Autodesk Inventor part; units mm, degrees
(part 5 of 7)
  arc A234 (19.9489, -1.9822) -> (19.5895, -1.8197) centre (17.1307, -7.7369) ccw projected
  arc A235 (20.3804, -2.2111) -> (19.9489, -1.9822) centre (16.6119, -8.7963) ccw projected
  arc A236 (20.3335, -2.6078) -> (20.3804, -2.2111) centre (0, 0) ccw projected
  arc A237 (19.8604, -2.7295) -> (20.3335, -2.6078) centre (18.2064, 4.6753) ccw projected
  arc A238 (19.473, -2.8036) -> (19.8604, -2.7295) centre (18.4635, 3.5241) ccw projected
  arc A239 (19.1652, -2.8435) -> (19.473, -2.8036) centre (18.6425, 2.4025) ccw projected
  arc A240 (19.1059, -3.2181) -> (19.1652, -2.8435) centre (0, 0) ccw projected
  arc A241 (19.3863, -3.3511) -> (19.1059, -3.2181) centre (16.9876, -8.0457) ccw projected
  arc A242 (19.7318, -3.5413) -> (19.3863, -3.3511) centre (16.4708, -9.0571) ccw projected
  arc A243 (20.1441, -3.8033) -> (19.7318, -3.5413) centre (15.8705, -10.0726) ccw projected
  arc A244 (20.0662, -4.1951) -> (20.1441, -3.8033) centre (0, 0) ccw projected
  arc A245 (19.585, -4.2793) -> (20.0662, -4.1951) centre (18.517, 3.2324) ccw projected
  arc A246 (19.193, -4.3228) -> (19.585, -4.2793) centre (18.6831, 2.0646) ccw projected
  arc A247 (18.883, -4.3384) -> (19.193, -4.3228) centre (18.7735, 0.9324) ccw projected
  arc A248 (18.7945, -4.7072) -> (18.883, -4.3384) centre (0, 0) ccw projected
  arc A249 (19.0636, -4.8618) -> (18.7945, -4.7072) centre (16.304, -9.3537) ccw projected
  arc A250 (19.3932, -5.0785) -> (19.0636, -4.8618) centre (15.7095, -10.3215) ccw projected
  arc A251 (19.7836, -5.372) -> (19.3932, -5.0785) centre (15.0313, -11.2867) ccw projected
  arc A252 (19.6752, -5.7565) -> (19.7836, -5.372) centre (0, 0) ccw projected
  arc A253 (19.1889, -5.8028) -> (19.6752, -5.7565) centre (18.7136, 1.7696) ccw projected
  arc A254 (18.7947, -5.8154) -> (19.1889, -5.8028) centre (18.7875, 0.5924) ccw projected
  arc A255 (18.4844, -5.8066) -> (18.7947, -5.8154) centre (18.7888, -0.5434) ccw projected
  arc A256 (18.3672, -6.1673) -> (18.4844, -5.8066) centre (0, 0) ccw projected
  arc A257 (18.6234, -6.3425) -> (18.3672, -6.1673) centre (15.5199, -10.6041) ccw projected
  arc A258 (18.9349, -6.5844) -> (18.6234, -6.3425) centre (14.8512, -11.5222) ccw projected
  arc A259 (19.3011, -6.9077) -> (18.9349, -6.5844) centre (14.0994, -12.4312) ccw projected
  arc A260 (19.1629, -7.2825) -> (19.3011, -6.9077) centre (0, 0) ccw projected
  arc A261 (18.6745, -7.2904) -> (19.1629, -7.2825) centre (18.7947, 0.2959) ccw projected
  arc A262 (18.2805, -7.272) -> (18.6745, -7.2904) centre (18.776, -0.8835) ccw projected
  arc A263 (17.9719, -7.2389) -> (18.2805, -7.272) centre (18.6882, -2.0159) ccw projected
  arc A264 (17.8267, -7.5893) -> (17.9719, -7.2389) centre (0, 0) ccw projected
  arc A265 (18.0684, -7.7842) -> (17.8267, -7.5893) centre (14.64, -11.7891) ccw projected
  arc A266 (18.36, -8.0497) -> (18.0684, -7.7842) centre (13.9014, -12.6519) ccw projected
  arc A267 (18.6997, -8.4007) -> (18.36, -8.0497) centre (13.0806, -13.4991) ccw projected
  arc A268 (18.5324, -8.7635) -> (18.6997, -8.4007) centre (0, 0) ccw projected
  arc A269 (18.0449, -8.7331) -> (18.5324, -8.7635) centre (18.76, -1.1796) ccw projected
  arc A270 (17.6536, -8.6839) -> (18.0449, -8.7331) centre (18.6488, -2.3539) ccw projected
  arc A271 (17.3485, -8.6267) -> (17.6536, -8.6839) centre (18.4724, -3.476) ccw projected
  arc A272 (17.1763, -8.9646) -> (17.3485, -8.6267) centre (0, 0) ccw projected
  arc A273 (17.4019, -9.1778) -> (17.1763, -8.9646) centre (13.6699, -12.9014) ccw projected
  arc A274 (17.6718, -9.4654) -> (17.4019, -9.1778) centre (12.8659, -13.7036) ccw projected
  arc A275 (17.9829, -9.842) -> (17.6718, -9.4654) centre (11.9812, -14.4838) ccw projected
  arc A276 (17.7877, -10.1905) -> (17.9829, -9.842) centre (0, 0) ccw projected
  arc A277 (17.3041, -10.122) -> (17.7877, -10.1905) centre (18.6096, -2.6478) ccw projected
  arc A278 (16.9178, -10.0422) -> (17.3041, -10.122) centre (18.4067, -3.8099) ccw projected
  arc A279 (16.6182, -9.9612) -> (16.9178, -10.0422) centre (18.1428, -4.9146) ccw projected
  arc A280 (16.42, -10.2846) -> (16.6182, -9.9612) centre (0, 0) ccw projected
  arc A281 (16.6282, -10.5148) -> (16.42, -10.2846) centre (12.6156, -13.9341) ccw projected
  arc A282 (16.8747, -10.8227) -> (16.6282, -10.5148) centre (11.7511, -14.6708) ccw projected
  arc A283 (17.1553, -11.2226) -> (16.8747, -10.8227) centre (10.8078, -15.3792) ccw projected
  arc A284 (16.9334, -11.5547) -> (17.1553, -11.2226) centre (0, 0) ccw projected
  arc A285 (16.4566, -11.4485) -> (16.9334, -11.5547) centre (18.3445, -4.0998) ccw projected
  arc A286 (16.0778, -11.3386) -> (16.4566, -11.4485) centre (18.051, -5.2423) ccw projected
  arc A287 (15.7854, -11.2344) -> (16.0778, -11.3386) centre (17.7012, -6.3229) ccw projected
  arc A288 (15.5625, -11.5412) -> (15.7854, -11.2344) centre (0, 0) ccw projected
  arc A289 (15.752, -11.7871) -> (15.5625, -11.5412) centre (11.4834, -14.881) ccw projected
  arc A290 (15.9735, -12.1134) -> (15.752, -11.7871) centre (10.5638, -15.5476) ccw projected
  arc A291 (16.2219, -12.534) -> (15.9735, -12.1134) centre (9.5679, -16.1798) ccw projected
  arc A292 (15.9746, -12.8477) -> (16.2219, -12.534) centre (0, 0) ccw projected
  arc A293 (15.5076, -12.7043) -> (15.9746, -12.8477) centre (17.9663, -5.5264) ccw projected
  arc A294 (15.1386, -12.5651) -> (15.5076, -12.7043) centre (17.5841, -6.6424) ccw projected
  arc A295 (14.8553, -12.4383) -> (15.1386, -12.5651) centre (17.1506, -7.6922) ccw projected
  arc A296 (14.609, -12.7266) -> (14.8553, -12.4383) centre (0, 0) ccw projected
  arc A297 (14.7786, -12.9866) -> (14.609, -12.7266) centre (10.2805, -15.7361) ccw projected
  arc A298 (14.9739, -13.3293) -> (14.7786, -12.9866) centre (9.3114, -16.3285) ccw projected
  arc A299 (15.1885, -13.7681) -> (14.9739, -13.3293) centre (8.2689, -16.8806) ccw projected
  arc A300 (14.9173, -14.0614) -> (15.1885, -13.7681) centre (0, 0) ccw projected
  arc A301 (14.463, -13.8819) -> (14.9173, -14.0614) centre (17.4773, -6.919) ccw projected
  arc A302 (14.1061, -13.7141) -> (14.463, -13.8819) centre (17.0087, -8.0015) ccw projected
  arc A303 (13.8336, -13.5655) -> (14.1061, -13.7141) centre (16.4942, -9.0141) ccw projected
  arc A304 (13.5655, -13.8336) -> (13.8336, -13.5655) centre (0, 0) ccw projected
  arc A305 (13.7141, -14.1061) -> (13.5655, -13.8336) centre (9.0141, -16.4942) ccw projected
  arc A306 (13.8819, -14.463) -> (13.7141, -14.1061) centre (8.0015, -17.0087) ccw projected
  arc A307 (14.0614, -14.9173) -> (13.8819, -14.463) centre (6.919, -17.4773) ccw projected
  arc A308 (13.7681, -15.1885) -> (14.0614, -14.9173) centre (0, 0) ccw projected
  arc A309 (13.3293, -14.9739) -> (13.7681, -15.1885) centre (16.8806, -8.2689) ccw projected
  arc A310 (12.9866, -14.7786) -> (13.3293, -14.9739) centre (16.3285, -9.3114) ccw projected
  arc A311 (12.7266, -14.609) -> (12.9866, -14.7786) centre (15.7361, -10.2805) ccw projected
  arc A312 (12.4383, -14.8553) -> (12.7266, -14.609) centre (0, 0) ccw projected
  arc A313 (12.5651, -15.1386) -> (12.4383, -14.8553) centre (7.6922, -17.1506) ccw projected
  arc A314 (12.7043, -15.5076) -> (12.5651, -15.1386) centre (6.6424, -17.5841) ccw projected
  arc A315 (12.8477, -15.9746) -> (12.7043, -15.5076) centre (5.5264, -17.9663) ccw projected
  arc A316 (12.534, -16.2219) -> (12.8477, -15.9746) centre (0, 0) ccw projected
  arc A317 (12.1134, -15.9735) -> (12.534, -16.2219) centre (16.1798, -9.5679) ccw projected
  arc A318 (11.7871, -15.752) -> (12.1134, -15.9735) centre (15.5476, -10.5638) ccw projected
  arc A319 (11.5412, -15.5625) -> (11.7871, -15.752) centre (14.881, -11.4834) ccw projected
  arc A320 (11.2344, -15.7854) -> (11.5412, -15.5625) centre (0, 0) ccw projected
  arc A321 (11.3386, -16.0778) -> (11.2344, -15.7854) centre (6.3229, -17.7012) ccw projected
  arc A322 (11.4485, -16.4566) -> (11.3386, -16.0778) centre (5.2423, -18.051) ccw projected
  arc A323 (11.5547, -16.9334) -> (11.4485, -16.4566) centre (4.0998, -18.3445) ccw projected
  arc A324 (11.2226, -17.1553) -> (11.5547, -16.9334) centre (0, 0) ccw projected
  arc A325 (10.8227, -16.8747) -> (11.2226, -17.1553) centre (15.3792, -10.8078) ccw projected
  arc A326 (10.5148, -16.6282) -> (10.8227, -16.8747) centre (14.6708, -11.7511) ccw projected
  arc A327 (10.2846, -16.42) -> (10.5148, -16.6282) centre (13.9341, -12.6156) ccw projected
  arc A328 (9.9612, -16.6182) -> (10.2846, -16.42) centre (0, 0) ccw projected
  arc A329 (10.0422, -16.9178) -> (9.9612, -16.6182) centre (4.9146, -18.1428) ccw projected
  arc A330 (10.122, -17.3041) -> (10.0422, -16.9178) centre (3.8099, -18.4067) ccw projected
  arc A331 (10.1905, -17.7877) -> (10.122, -17.3041) centre (2.6478, -18.6096) ccw projected
  arc A332 (9.842, -17.9829) -> (10.1905, -17.7877) centre (0, 0) ccw projected
  arc A333 (9.4654, -17.6718) -> (9.842, -17.9829) centre (14.4838, -11.9812) ccw projected
  arc A334 (9.1778, -17.4019) -> (9.4654, -17.6718) centre (13.7036, -12.8659) ccw projected
  arc A335 (8.9646, -17.1763) -> (9.1778, -17.4019) centre (12.9014, -13.6699) ccw projected
  arc A336 (8.6267, -17.3485) -> (8.9646, -17.1763) centre (0, 0) ccw projected
  arc A337 (8.6839, -17.6536) -> (8.6267, -17.3485) centre (3.476, -18.4724) ccw projected
  arc A338 (8.7331, -18.0449) -> (8.6839, -17.6536) centre (2.3539, -18.6488) ccw projected
  arc A339 (8.7635, -18.5324) -> (8.7331, -18.0449) centre (1.1796, -18.76) ccw projected
  arc A340 (8.4007, -18.6997) -> (8.7635, -18.5324) centre (0, 0) ccw projected
  arc A341 (8.0497, -18.36) -> (8.4007, -18.6997) centre (13.4991, -13.0806) ccw projected
  arc A342 (7.7842, -18.0684) -> (8.0497, -18.36) centre (12.6519, -13.9014) ccw projected
  arc A343 (7.5893, -17.8267) -> (7.7842, -18.0684) centre (11.7891, -14.64) ccw projected
  arc A344 (7.2389, -17.9719) -> (7.5893, -17.8267) centre (0, 0) ccw projected
  arc A345 (7.272, -18.2805) -> (7.2389, -17.9719) centre (2.0159, -18.6882) ccw projected
  arc A346 (7.2904, -18.6745) -> (7.272, -18.2805) centre (0.8835, -18.776) ccw projected
  arc A347 (7.2825, -19.1629) -> (7.2904, -18.6745) centre (-0.2959, -18.7947) ccw projected
  arc A348 (6.9077, -19.3011) -> (7.2825, -19.1629) centre (0, 0) ccw projected
  arc A349 (6.5844, -18.9349) -> (6.9077, -19.3011) centre (12.4312, -14.0994) ccw projected
  arc A350 (6.3425, -18.6234) -> (6.5844, -18.9349) centre (11.5222, -14.8512) ccw projected
  arc A351 (6.1673, -18.3672) -> (6.3425, -18.6234) centre (10.6041, -15.5199) ccw projected
  arc A352 (5.8066, -18.4844) -> (6.1673, -18.3672) centre (0, 0) ccw projected
  arc A353 (5.8154, -18.7947) -> (5.8066, -18.4844) centre (0.5434, -18.7888) ccw projected
  arc A354 (5.8028, -19.1889) -> (5.8154, -18.7947) centre (-0.5924, -18.7875) ccw projected
  arc A355 (5.7565, -19.6752) -> (5.8028, -19.1889) centre (-1.7696, -18.7136) ccw projected
  arc A356 (5.372, -19.7836) -> (5.7565, -19.6752) centre (0, 0) ccw projected
  arc A357 (5.0785, -19.3932) -> (5.372, -19.7836) centre (11.2867, -15.0313) ccw projected
  arc A358 (4.8618, -19.0636) -> (5.0785, -19.3932) centre (10.3215, -15.7095) ccw projected
  arc A359 (4.7072, -18.7945) -> (4.8618, -19.0636) centre (9.3537, -16.304) ccw projected
  arc A360 (4.3384, -18.883) -> (4.7072, -18.7945) centre (0, 0) ccw projected
  arc A361 (4.3228, -19.193) -> (4.3384, -18.883) centre (-0.9324, -18.7735) ccw projected
  arc A362 (4.2793, -19.585) -> (4.3228, -19.193) centre (-2.0646, -18.6831) ccw projected
  arc A363 (4.1951, -20.0662) -> (4.2793, -19.585) centre (-3.2324, -18.517) ccw projected
  arc A364 (3.8033, -20.1441) -> (4.1951, -20.0662) centre (0, 0) ccw projected
  arc A365 (3.5413, -19.7318) -> (3.8033, -20.1441) centre (10.0726, -15.8705) ccw projected
  arc A366 (3.3511, -19.3863) -> (3.5413, -19.7318) centre (9.0571, -16.4708) ccw projected
  arc A367 (3.2181, -19.1059) -> (3.3511, -19.3863) centre (8.0457, -16.9876) ccw projected
  arc A368 (2.8435, -19.1652) -> (3.2181, -19.1059) centre (0, 0) ccw projected
  arc A369 (2.8036, -19.473) -> (2.8435, -19.1652) centre (-2.4025, -18.6425) ccw projected
  arc A370 (2.7295, -19.8604) -> (2.8036, -19.473) centre (-3.5241, -18.4635) ccw projected
  arc A371 (2.6078, -20.3335) -> (2.7295, -19.8604) centre (-4.6753, -18.2064) ccw projected
  arc A372 (2.2111, -20.3804) -> (2.6078, -20.3335) centre (0, 0) ccw projected
  arc A373 (1.9822, -19.9489) -> (2.2111, -20.3804) centre (8.7963, -16.6119) ccw projected
  arc A374 (1.8197, -19.5895) -> (1.9822, -19.9489) centre (7.7369, -17.1307) ccw projected
  arc A375 (1.7091, -19.2995) -> (1.8197, -19.5895) centre (6.6881, -17.5665) ccw projected
  arc A376 (1.331, -19.3292) -> (1.7091, -19.2995) centre (0, 0) ccw projected
  arc A377 (1.2671, -19.633) -> (1.331, -19.3292) centre (-3.8577, -18.3965) ccw projected
  arc A378 (1.1629, -20.0133) -> (1.2671, -19.633) centre (-4.9618, -18.1301) ccw projected
  arc A379 (1.0044, -20.4754) -> (1.1629, -20.0133) centre (-6.0894, -17.7834) ccw projected
  arc A380 (0.6052, -20.4911) -> (1.0044, -20.4754) centre (0, 0) ccw projected
  arc A381 (0.4109, -20.0429) -> (0.6052, -20.4911) centre (7.4658, -17.2508) ccw projected
  arc A382 (0.2771, -19.6719) -> (0.4109, -20.0429) centre (6.369, -17.6849) ccw projected
  arc A383 (0.1896, -19.3741) -> (0.2771, -19.6719) centre (5.2892, -18.0371) ccw projected
  arc A384 (-0.1896, -19.3741) -> (0.1896, -19.3741) centre (0, 0) ccw projected
  arc A385 (-0.2771, -19.6719) -> (-0.1896, -19.3741) centre (-5.2892, -18.0371) ccw projected
  arc A386 (-0.4109, -20.0429) -> (-0.2771, -19.6719) centre (-6.369, -17.6849) ccw projected
  arc A387 (-0.6052, -20.4911) -> (-0.4109, -20.0429) centre (-7.4658, -17.2508) ccw projected
  arc A388 (-1.0044, -20.4754) -> (-0.6052, -20.4911) centre (0, 0) ccw projected
  arc A389 (-1.1629, -20.0133) -> (-1.0044, -20.4754) centre (6.0894, -17.7834) ccw projected
  arc A390 (-1.2671, -19.633) -> (-1.1629, -20.0133) centre (4.9618, -18.1301) ccw projected
  arc A391 (-1.331, -19.3292) -> (-1.2671, -19.633) centre (3.8577, -18.3965) ccw projected
  arc A392 (-1.7091, -19.2995) -> (-1.331, -19.3292) centre (0, 0) ccw projected
  arc A393 (-1.8197, -19.5895) -> (-1.7091, -19.2995) centre (-6.6881, -17.5665) ccw projected
  arc A394 (-1.9822, -19.9489) -> (-1.8197, -19.5895) centre (-7.7369, -17.1307) ccw projected
  arc A395 (-2.2111, -20.3804) -> (-1.9822, -19.9489) centre (-8.7963, -16.6119) ccw projected
  arc A396 (-2.6078, -20.3335) -> (-2.2111, -20.3804) centre (0, 0) ccw projected
  arc A397 (-2.7295, -19.8604) -> (-2.6078, -20.3335) centre (4.6753, -18.2064) ccw projected
  arc A398 (-2.8036, -19.473) -> (-2.7295, -19.8604) centre (3.5241, -18.4635) ccw projected
  arc A399 (-2.8435, -19.1652) -> (-2.8036, -19.473) centre (2.4025, -18.6425) ccw projected
  arc A400 (-3.2181, -19.1059) -> (-2.8435, -19.1652) centre (0, 0) ccw projected
  arc A401 (-3.3511, -19.3863) -> (-3.2181, -19.1059) centre (-8.0457, -16.9876) ccw projected
  arc A402 (-3.5413, -19.7318) -> (-3.3511, -19.3863) centre (-9.0571, -16.4708) ccw projected
  arc A403 (-3.8033, -20.1441) -> (-3.5413, -19.7318) centre (-10.0726, -15.8705) ccw projected
  arc A404 (-4.1951, -20.0662) -> (-3.8033, -20.1441) centre (0, 0) ccw projected
  arc A405 (-4.2793, -19.585) -> (-4.1951, -20.0662) centre (3.2324, -18.517) ccw projected
  arc A406 (-4.3228, -19.193) -> (-4.2793, -19.585) centre (2.0646, -18.6831) ccw projected
  arc A407 (-4.3384, -18.883) -> (-4.3228, -19.193) centre (0.9324, -18.7735) ccw projected
  arc A408 (-4.7072, -18.7945) -> (-4.3384, -18.883) centre (0, 0) ccw projected
  arc A409 (-4.8618, -19.0636) -> (-4.7072, -18.7945) centre (-9.3537, -16.304) ccw projected
  arc A410 (-5.0785, -19.3932) -> (-4.8618, -19.0636) centre (-10.3215, -15.7095) ccw projected
  arc A411 (-5.372, -19.7836) -> (-5.0785, -19.3932) centre (-11.2867, -15.0313) ccw projected
  arc A412 (-5.7565, -19.6752) -> (-5.372, -19.7836) centre (0, 0) ccw projected
  arc A413 (-5.8028, -19.1889) -> (-5.7565, -19.6752) centre (1.7696, -18.7136) ccw projected
  arc A414 (-5.8154, -18.7947) -> (-5.8028, -19.1889) centre (0.5924, -18.7875) ccw projected
  arc A415 (-5.8066, -18.4844) -> (-5.8154, -18.7947) centre (-0.5434, -18.7888) ccw projected
  arc A416 (-6.1673, -18.3672) -> (-5.8066, -18.4844) centre (0, 0) ccw projected
  arc A417 (-6.3425, -18.6234) -> (-6.1673, -18.3672) centre (-10.6041, -15.5199) ccw projected
  arc A418 (-6.5844, -18.9349) -> (-6.3425, -18.6234) centre (-11.5222, -14.8512) ccw projected
  arc A419 (-6.9077, -19.3011) -> (-6.5844, -18.9349) centre (-12.4312, -14.0994) ccw projected
  arc A420 (-7.2825, -19.1629) -> (-6.9077, -19.3011) centre (0, 0) ccw projected
  arc A421 (-7.2904, -18.6745) -> (-7.2825, -19.1629) centre (0.2959, -18.7947) ccw projected
  arc A422 (-7.272, -18.2805) -> (-7.2904, -18.6745) centre (-0.8835, -18.776) ccw projected
  arc A423 (-7.2389, -17.9719) -> (-7.272, -18.2805) centre (-2.0159, -18.6882) ccw projected
  arc A424 (-7.5893, -17.8267) -> (-7.2389, -17.9719) centre (0, 0) ccw projected
  arc A425 (-7.7842, -18.0684) -> (-7.5893, -17.8267) centre (-11.7891, -14.64) ccw projected
  arc A426 (-8.0497, -18.36) -> (-7.7842, -18.0684) centre (-12.6519, -13.9014) ccw projected
  arc A427 (-8.4007, -18.6997) -> (-8.0497, -18.36) centre (-13.4991, -13.0806) ccw projected
  arc A428 (-8.7635, -18.5324) -> (-8.4007, -18.6997) centre (0, 0) ccw projected
  arc A429 (-8.7331, -18.0449) -> (-8.7635, -18.5324) centre (-1.1796, -18.76) ccw projected
  arc A430 (-8.6839, -17.6536) -> (-8.7331, -18.0449) centre (-2.3539, -18.6488) ccw projected
  arc A431 (-8.6267, -17.3485) -> (-8.6839, -17.6536) centre (-3.476, -18.4724) ccw projected
  arc A432 (-8.9646, -17.1763) -> (-8.6267, -17.3485) centre (0, 0) ccw projected
  arc A433 (-9.1778, -17.4019) -> (-8.9646, -17.1763) centre (-12.9014, -13.6699) ccw projected
  arc A434 (-9.4654, -17.6718) -> (-9.1778, -17.4019) centre (-13.7036, -12.8659) ccw projected
  arc A435 (-9.842, -17.9829) -> (-9.4654, -17.6718) centre (-14.4838, -11.9812) ccw projected
  arc A436 (-10.1905, -17.7877) -> (-9.842, -17.9829) centre (0, 0) ccw projected
  arc A437 (-10.122, -17.3041) -> (-10.1905, -17.7877) centre (-2.6478, -18.6096) ccw projected
  arc A438 (-10.0422, -16.9178) -> (-10.122, -17.3041) centre (-3.8099, -18.4067) ccw projected
  arc A439 (-9.9612, -16.6182) -> (-10.0422, -16.9178) centre (-4.9146, -18.1428) ccw projected
  arc A440 (-10.2846, -16.42) -> (-9.9612, -16.6182) centre (0, 0) ccw projected
  arc A441 (-10.5148, -16.6282) -> (-10.2846, -16.42) centre (-13.9341, -12.6156) ccw projected
  arc A442 (-10.8227, -16.8747) -> (-10.5148, -16.6282) centre (-14.6708, -11.7511) ccw projected
  arc A443 (-11.2226, -17.1553) -> (-10.8227, -16.8747) centre (-15.3792, -10.8078) ccw projected
  arc A444 (-11.5547, -16.9334) -> (-11.2226, -17.1553) centre (0, 0) ccw projected
  arc A445 (-11.4485, -16.4566) -> (-11.5547, -16.9334) centre (-4.0998, -18.3445) ccw projected
  arc A446 (-11.3386, -16.0778) -> (-11.4485, -16.4566) centre (-5.2423, -18.051) ccw projected
  arc A447 (-11.2344, -15.7854) -> (-11.3386, -16.0778) centre (-6.3229, -17.7012) ccw projected
  arc A448 (-11.5412, -15.5625) -> (-11.2344, -15.7854) centre (0, 0) ccw projected
  arc A449 (-11.7871, -15.752) -> (-11.5412, -15.5625) centre (-14.881, -11.4834) ccw projected
  arc A450 (-12.1134, -15.9735) -> (-11.7871, -15.752) centre (-15.5476, -10.5638) ccw projected
  arc A451 (-12.534, -16.2219) -> (-12.1134, -15.9735) centre (-16.1798, -9.5679) ccw projected
  arc A452 (-12.8477, -15.9746) -> (-12.534, -16.2219) centre (0, 0) ccw projected
  arc A453 (-12.7043, -15.5076) -> (-12.8477, -15.9746) centre (-5.5264, -17.9663) ccw projected
  arc A454 (-12.5651, -15.1386) -> (-12.7043, -15.5076) centre (-6.6424, -17.5841) ccw projected
  arc A455 (-12.4383, -14.8553) -> (-12.5651, -15.1386) centre (-7.6922, -17.1506) ccw projected
  arc A456 (-12.7266, -14.609) -> (-12.4383, -14.8553) centre (0, 0) ccw projected
  arc A457 (-12.9866, -14.7786) -> (-12.7266, -14.609) centre (-15.7361, -10.2805) ccw projected
  arc A458 (-13.3293, -14.9739) -> (-12.9866, -14.7786) centre (-16.3285, -9.3114) ccw projected
  arc A459 (-13.7681, -15.1885) -> (-13.3293, -14.9739) centre (-16.8806, -8.2689) ccw projected
  arc A460 (-14.0614, -14.9173) -> (-13.7681, -15.1885) centre (0, 0) ccw projected
  arc A461 (-13.8819, -14.463) -> (-14.0614, -14.9173) centre (-6.919, -17.4773) ccw projected
  arc A462 (-13.7141, -14.1061) -> (-13.8819, -14.463) centre (-8.0015, -17.0087) ccw projected
  arc A463 (-13.5655, -13.8336) -> (-13.7141, -14.1061) centre (-9.0141, -16.4942) ccw projected
  arc A464 (-13.8336, -13.5655) -> (-13.5655, -13.8336) centre (0, 0) ccw projected
  arc A465 (-14.1061, -13.7141) -> (-13.8336, -13.5655) centre (-16.4942, -9.0141) ccw projected
  arc A466 (-14.463, -13.8819) -> (-14.1061, -13.7141) centre (-17.0087, -8.0015) ccw projected
  arc A467 (-14.9173, -14.0614) -> (-14.463, -13.8819) centre (-17.4773, -6.919) ccw projected
  arc A468 (-15.1885, -13.7681) -> (-14.9173, -14.0614) centre (0, 0) ccw projected
  arc A469 (-14.9739, -13.3293) -> (-15.1885, -13.7681) centre (-8.2689, -16.8806) ccw projected
  arc A470 (-14.7786, -12.9866) -> (-14.9739, -13.3293) centre (-9.3114, -16.3285) ccw projected
  arc A471 (-14.609, -12.7266) -> (-14.7786, -12.9866) centre (-10.2805, -15.7361) ccw projected
  arc A472 (-14.8553, -12.4383) -> (-14.609, -12.7266) centre (0, 0) ccw projected
  arc A473 (-15.1386, -12.5651) -> (-14.8553, -12.4383) centre (-17.1506, -7.6922) ccw projected
  arc A474 (-15.5076, -12.7043) -> (-15.1386, -12.5651) centre (-17.5841, -6.6424) ccw projected
  arc A475 (-15.9746, -12.8477) -> (-15.5076, -12.7043) centre (-17.9663, -5.5264) ccw projected
  arc A476 (-16.2219, -12.534) -> (-15.9746, -12.8477) centre (0, 0) ccw projected
  arc A477 (-15.9735, -12.1134) -> (-16.2219, -12.534) centre (-9.5679, -16.1798) ccw projected
  arc A478 (-15.752, -11.7871) -> (-15.9735, -12.1134) centre (-10.5638, -15.5476) ccw projected
  arc A479 (-15.5625, -11.5412) -> (-15.752, -11.7871) centre (-11.4834, -14.881) ccw projected
  arc A480 (-15.7854, -11.2344) -> (-15.5625, -11.5412) centre (0, 0) ccw projected
  arc A481 (-16.0778, -11.3386) -> (-15.7854, -11.2344) centre (-17.7012, -6.3229) ccw projected
  arc A482 (-16.4566, -11.4485) -> (-16.0778, -11.3386) centre (-18.051, -5.2423) ccw projected
  arc A483 (-16.9334, -11.5547) -> (-16.4566, -11.4485) centre (-18.3445, -4.0998) ccw projected
  arc A484 (-17.1553, -11.2226) -> (-16.9334, -11.5547) centre (0, 0) ccw projected
  arc A485 (-16.8747, -10.8227) -> (-17.1553, -11.2226) centre (-10.8078, -15.3792) ccw projected
  arc A486 (-16.6282, -10.5148) -> (-16.8747, -10.8227) centre (-11.7511, -14.6708) ccw projected
  arc A487 (-16.42, -10.2846) -> (-16.6282, -10.5148) centre (-12.6156, -13.9341) ccw projected
  arc A488 (-16.6182, -9.9612) -> (-16.42, -10.2846) centre (0, 0) ccw projected
  arc A489 (-16.9178, -10.0422) -> (-16.6182, -9.9612) centre (-18.1428, -4.9146) ccw projected
  arc A490 (-17.3041, -10.122) -> (-16.9178, -10.0422) centre (-18.4067, -3.8099) ccw projected
  arc A491 (-17.7877, -10.1905) -> (-17.3041, -10.122) centre (-18.6096, -2.6478) ccw projected
  arc A492 (-17.9829, -9.842) -> (-17.7877, -10.1905) centre (0, 0) ccw projected
  arc A493 (-17.6718, -9.4654) -> (-17.9829, -9.842) centre (-11.9812, -14.4838) ccw projected
  arc A494 (-17.4019, -9.1778) -> (-17.6718, -9.4654) centre (-12.8659, -13.7036) ccw projected
  arc A495 (-17.1763, -8.9646) -> (-17.4019, -9.1778) centre (-13.6699, -12.9014) ccw projected
  arc A496 (-17.3485, -8.6267) -> (-17.1763, -8.9646) centre (0, 0) ccw projected
  arc A497 (-17.6536, -8.6839) -> (-17.3485, -8.6267) centre (-18.4724, -3.476) ccw projected
  arc A498 (-18.0449, -8.7331) -> (-17.6536, -8.6839) centre (-18.6488, -2.3539) ccw projected
  arc A499 (-18.5324, -8.7635) -> (-18.0449, -8.7331) centre (-18.76, -1.1796) ccw projected
  arc A500 (-18.6997, -8.4007) -> (-18.5324, -8.7635) centre (0, 0) ccw projected
  arc A501 (-18.36, -8.0497) -> (-18.6997, -8.4007) centre (-13.0806, -13.4991) ccw projected
  arc A502 (-18.0684, -7.7842) -> (-18.36, -8.0497) centre (-13.9014, -12.6519) ccw projected
  arc A503 (-17.8267, -7.5893) -> (-18.0684, -7.7842) centre (-14.64, -11.7891) ccw projected
  arc A504 (-17.9719, -7.2389) -> (-17.8267, -7.5893) centre (0, 0) ccw projected
  arc A505 (-18.2805, -7.272) -> (-17.9719, -7.2389) centre (-18.6882, -2.0159) ccw projected
  arc A506 (-18.6745, -7.2904) -> (-18.2805, -7.272) centre (-18.776, -0.8835) ccw projected
  arc A507 (-19.1629, -7.2825) -> (-18.6745, -7.2904) centre (-18.7947, 0.2959) ccw projected
  arc A508 (-19.3011, -6.9077) -> (-19.1629, -7.2825) centre (0, 0) ccw projected
  arc A509 (-18.9349, -6.5844) -> (-19.3011, -6.9077) centre (-14.0994, -12.4312) ccw projected
  arc A510 (-18.6234, -6.3425) -> (-18.9349, -6.5844) centre (-14.8512, -11.5222) ccw projected
  arc A511 (-18.3672, -6.1673) -> (-18.6234, -6.3425) centre (-15.5199, -10.6041) ccw projected
  arc A512 (-18.4844, -5.8066) -> (-18.3672, -6.1673) centre (0, 0) ccw projected
  arc A513 (-18.7947, -5.8154) -> (-18.4844, -5.8066) centre (-18.7888, -0.5434) ccw projected
  arc A514 (-19.1889, -5.8028) -> (-18.7947, -5.8154) centre (-18.7875, 0.5924) ccw projected
  arc A515 (-19.6752, -5.7565) -> (-19.1889, -5.8028) centre (-18.7136, 1.7696) ccw projected
  arc A516 (-19.7836, -5.372) -> (-19.6752, -5.7565) centre (0, 0) ccw projected
  arc A517 (-19.3932, -5.0785) -> (-19.7836, -5.372) centre (-15.0313, -11.2867) ccw projected
  arc A518 (-19.0636, -4.8618) -> (-19.3932, -5.0785) centre (-15.7095, -10.3215) ccw projected
  arc A519 (-18.7945, -4.7072) -> (-19.0636, -4.8618) centre (-16.304, -9.3537) ccw projected
  arc A520 (-18.883, -4.3384) -> (-18.7945, -4.7072) centre (0, 0) ccw projected
  arc A521 (-19.193, -4.3228) -> (-18.883, -4.3384) centre (-18.7735, 0.9324) ccw projected
  arc A522 (-19.585, -4.2793) -> (-19.193, -4.3228) centre (-18.6831, 2.0646) ccw projected
  arc A523 (-20.0662, -4.1951) -> (-19.585, -4.2793) centre (-18.517, 3.2324) ccw projected
  arc A524 (-20.1441, -3.8033) -> (-20.0662, -4.1951) centre (0, 0) ccw projected
  arc A525 (-19.7318, -3.5413) -> (-20.1441, -3.8033) centre (-15.8705, -10.0726) ccw projected
  arc A526 (-19.3863, -3.3511) -> (-19.7318, -3.5413) centre (-16.4708, -9.0571) ccw projected
  arc A527 (-19.1059, -3.2181) -> (-19.3863, -3.3511) centre (-16.9876, -8.0457) ccw projected
  arc A528 (-19.1652, -2.8435) -> (-19.1059, -3.2181) centre (0, 0) ccw projected
  arc A529 (-19.473, -2.8036) -> (-19.1652, -2.8435) centre (-18.6425, 2.4025) ccw projected
  arc A530 (-19.8604, -2.7295) -> (-19.473, -2.8036) centre (-18.4635, 3.5241) ccw projected
  arc A531 (-20.3335, -2.6078) -> (-19.8604, -2.7295) centre (-18.2064, 4.6753) ccw projected
  arc A532 (-20.3804, -2.2111) -> (-20.3335, -2.6078) centre (0, 0) ccw projected
  arc A533 (-19.9489, -1.9822) -> (-20.3804, -2.2111) centre (-16.6119, -8.7963) ccw projected
  arc A534 (-19.5895, -1.8197) -> (-19.9489, -1.9822) centre (-17.1307, -7.7369) ccw projected
  arc A535 (-19.2995, -1.7091) -> (-19.5895, -1.8197) centre (-17.5665, -6.6881) ccw projected
  arc A536 (-19.3292, -1.331) -> (-19.2995, -1.7091) centre (0, 0) ccw projected
  arc A537 (-19.633, -1.2671) -> (-19.3292, -1.331) centre (-18.3965, 3.8577) ccw projected
  arc A538 (-20.0133, -1.1629) -> (-19.633, -1.2671) centre (-18.1301, 4.9618) ccw projected
  arc A539 (-20.4754, -1.0044) -> (-20.0133, -1.1629) centre (-17.7834, 6.0894) ccw projected
  arc A540 (-20.4911, -0.6052) -> (-20.4754, -1.0044) centre (0, 0) ccw projected
  arc A541 (-20.0429, -0.4109) -> (-20.4911, -0.6052) centre (-17.2508, -7.4658) ccw projected
  arc A542 (-19.6719, -0.2771) -> (-20.0429, -0.4109) centre (-17.6849, -6.369) ccw projected
  arc A543 (-19.3741, -0.1896) -> (-19.6719, -0.2771) centre (-18.0371, -5.2892) ccw projected
  arc A544 (-19.3741, 0.1896) -> (-19.3741, -0.1896) centre (0, 0) ccw projected
  arc A545 (-19.6719, 0.2771) -> (-19.3741, 0.1896) centre (-18.0371, 5.2892) ccw projected
  arc A546 (-20.0429, 0.4109) -> (-19.6719, 0.2771) centre (-17.6849, 6.369) ccw projected
  arc A547 (-20.4911, 0.6052) -> (-20.0429, 0.4109) centre (-17.2508, 7.4658) ccw projected
  arc A548 (-20.4754, 1.0044) -> (-20.4911, 0.6052) centre (0, 0) ccw projected
  arc A549 (-20.0133, 1.1629) -> (-20.4754, 1.0044) centre (-17.7834, -6.0894) ccw projected
  arc A550 (-19.633, 1.2671) -> (-20.0133, 1.1629) centre (-18.1301, -4.9618) ccw projected
  arc A551 (-19.3292, 1.331) -> (-19.633, 1.2671) centre (-18.3965, -3.8577) ccw projected
  arc A552 (-19.2995, 1.7091) -> (-19.3292, 1.331) centre (0, 0) ccw projected
  arc A553 (-19.5895, 1.8197) -> (-19.2995, 1.7091) centre (-17.5665, 6.6881) ccw projected
  arc A554 (-19.9489, 1.9822) -> (-19.5895, 1.8197) centre (-17.1307, 7.7369) ccw projected
  arc A555 (-20.3804, 2.2111) -> (-19.9489, 1.9822) centre (-16.6119, 8.7963) ccw projected
  arc A556 (-20.3335, 2.6078) -> (-20.3804, 2.2111) centre (0, 0) ccw projected
  arc A557 (-19.8604, 2.7295) -> (-20.3335, 2.6078) centre (-18.2064, -4.6753) ccw projected
  arc A558 (-19.473, 2.8036) -> (-19.8604, 2.7295) centre (-18.4635, -3.5241) ccw projected
  arc A559 (-19.1652, 2.8435) -> (-19.473, 2.8036) centre (-18.6425, -2.4025) ccw projected
  arc A560 (-19.1059, 3.2181) -> (-19.1652, 2.8435) centre (0, 0) ccw projected
  arc A561 (-19.3863, 3.3511) -> (-19.1059, 3.2181) centre (-16.9876, 8.0457) ccw projected
  arc A562 (-19.7318, 3.5413) -> (-19.3863, 3.3511) centre (-16.4708, 9.0571) ccw projected
  arc A563 (-20.1441, 3.8033) -> (-19.7318, 3.5413) centre (-15.8705, 10.0726) ccw projected
  arc A564 (-20.0662, 4.1951) -> (-20.1441, 3.8033) centre (0, 0) ccw projected
  arc A565 (-19.585, 4.2793) -> (-20.0662, 4.1951) centre (-18.517, -3.2324) ccw projected
  arc A566 (-19.193, 4.3228) -> (-19.585, 4.2793) centre (-18.6831, -2.0646) ccw projected
  arc A567 (-18.883, 4.3384) -> (-19.193, 4.3228) centre (-18.7735, -0.9324) ccw projected
  arc A568 (-18.7945, 4.7072) -> (-18.883, 4.3384) centre (0, 0) ccw projected
  arc A569 (-19.0636, 4.8618) -> (-18.7945, 4.7072) centre (-16.304, 9.3537) ccw projected
  arc A570 (-19.3932, 5.0785) -> (-19.0636, 4.8618) centre (-15.7095, 10.3215) ccw projected
  arc A571 (-19.7836, 5.372) -> (-19.3932, 5.0785) centre (-15.0313, 11.2867) ccw projected
  arc A572 (-19.6752, 5.7565) -> (-19.7836, 5.372) centre (0, 0) ccw projected
  arc A573 (-19.1889, 5.8028) -> (-19.6752, 5.7565) centre (-18.7136, -1.7696) ccw projected
  arc A574 (-18.7947, 5.8154) -> (-19.1889, 5.8028) centre (-18.7875, -0.5924) ccw projected
  arc A575 (-18.4844, 5.8066) -> (-18.7947, 5.8154) centre (-18.7888, 0.5434) ccw projected
  arc A576 (-18.3672, 6.1673) -> (-18.4844, 5.8066) centre (0, 0) ccw projected
  arc A577 (-18.6234, 6.3425) -> (-18.3672, 6.1673) centre (-15.5199, 10.6041) ccw projected
  arc A578 (-18.9349, 6.5844) -> (-18.6234, 6.3425) centre (-14.8512, 11.5222) ccw projected
  arc A579 (-19.3011, 6.9077) -> (-18.9349, 6.5844) centre (-14.0994, 12.4312) ccw projected
  arc A580 (-19.1629, 7.2825) -> (-19.3011, 6.9077) centre (0, 0) ccw projected
  arc A581 (-18.6745, 7.2904) -> (-19.1629, 7.2825) centre (-18.7947, -0.2959) ccw projected
  arc A582 (-18.2805, 7.272) -> (-18.6745, 7.2904) centre (-18.776, 0.8835) ccw projected
  arc A583 (-17.9719, 7.2389) -> (-18.2805, 7.272) centre (-18.6882, 2.0159) ccw projected
  arc A584 (-17.8267, 7.5893) -> (-17.9719, 7.2389) centre (0, 0) ccw projected
  arc A585 (-18.0684, 7.7842) -> (-17.8267, 7.5893) centre (-14.64, 11.7891) ccw projected
  arc A586 (-18.36, 8.0497) -> (-18.0684, 7.7842) centre (-13.9014, 12.6519) ccw projected
  arc A587 (-18.6997, 8.4007) -> (-18.36, 8.0497) centre (-13.0806, 13.4991) ccw projected
  arc A588 (-18.5324, 8.7635) -> (-18.6997, 8.4007) centre (0, 0) ccw projected
  arc A589 (-18.0449, 8.7331) -> (-18.5324, 8.7635) centre (-18.76, 1.1796) ccw projected
  arc A590 (-17.6536, 8.6839) -> (-18.0449, 8.7331) centre (-18.6488, 2.3539) ccw projected
  arc A591 (-17.3485, 8.6267) -> (-17.6536, 8.6839) centre (-18.4724, 3.476) ccw projected
  arc A592 (-17.1763, 8.9646) -> (-17.3485, 8.6267) centre (0, 0) ccw projected
  arc A593 (-17.4019, 9.1778) -> (-17.1763, 8.9646) centre (-13.6699, 12.9014) ccw projected
  arc A594 (-17.6718, 9.4654) -> (-17.4019, 9.1778) centre (-12.8659, 13.7036) ccw projected
  arc A595 (-17.9829, 9.842) -> (-17.6718, 9.4654) centre (-11.9812, 14.4838) ccw projected
  arc A596 (-17.7877, 10.1905) -> (-17.9829, 9.842) centre (0, 0) ccw projected
  arc A597 (-17.3041, 10.122) -> (-17.7877, 10.1905) centre (-18.6096, 2.6478) ccw projected
  arc A598 (-16.9178, 10.0422) -> (-17.3041, 10.122) centre (-18.4067, 3.8099) ccw projected
  arc A599 (-16.6182, 9.9612) -> (-16.9178, 10.0422) centre (-18.1428, 4.9146) ccw projected
  arc A600 (-16.42, 10.2846) -> (-16.6182, 9.9612) centre (0, 0) ccw projected
  arc A601 (-16.6282, 10.5148) -> (-16.42, 10.2846) centre (-12.6156, 13.9341) ccw projected
  arc A602 (-16.8747, 10.8227) -> (-16.6282, 10.5148) centre (-11.7511, 14.6708) ccw projected
  arc A603 (-17.1553, 11.2226) -> (-16.8747, 10.8227) centre (-10.8078, 15.3792) ccw projected
  arc A604 (-16.9334, 11.5547) -> (-17.1553, 11.2226) centre (0, 0) ccw projected
  arc A605 (-16.4566, 11.4485) -> (-16.9334, 11.5547) centre (-18.3445, 4.0998) ccw projected
  arc A606 (-16.0778, 11.3386) -> (-16.4566, 11.4485) centre (-18.051, 5.2423) ccw projected
  arc A607 (-15.7854, 11.2344) -> (-16.0778, 11.3386) centre (-17.7012, 6.3229) ccw projected
  arc A608 (-15.5625, 11.5412) -> (-15.7854, 11.2344) centre (0, 0) ccw projected
  arc A609 (-15.752, 11.7871) -> (-15.5625, 11.5412) centre (-11.4834, 14.881) ccw projected
  arc A610 (-15.9735, 12.1134) -> (-15.752, 11.7871) centre (-10.5638, 15.5476) ccw projected
  arc A611 (-16.2219, 12.534) -> (-15.9735, 12.1134) centre (-9.5679, 16.1798) ccw projected
  arc A612 (-15.9746, 12.8477) -> (-16.2219, 12.534) centre (0, 0) ccw projected
  arc A613 (-15.5076, 12.7043) -> (-15.9746, 12.8477) centre (-17.9663, 5.5264) ccw projected
  arc A614 (-15.1386, 12.5651) -> (-15.5076, 12.7043) centre (-17.5841, 6.6424) ccw projected
  arc A615 (-14.8553, 12.4383) -> (-15.1386, 12.5651) centre (-17.1506, 7.6922) ccw projected
  arc A616 (-14.609, 12.7266) -> (-14.8553, 12.4383) centre (0, 0) ccw projected
  arc A617 (-14.7786, 12.9866) -> (-14.609, 12.7266) centre (-10.2805, 15.7361) ccw projected
  arc A618 (-14.9739, 13.3293) -> (-14.7786, 12.9866) centre (-9.3114, 16.3285) ccw projected
  arc A619 (-15.1885, 13.7681) -> (-14.9739, 13.3293) centre (-8.2689, 16.8806) ccw projected
  arc A620 (-14.9173, 14.0614) -> (-15.1885, 13.7681) centre (0, 0) ccw projected
  arc A621 (-14.463, 13.8819) -> (-14.9173, 14.0614) centre (-17.4773, 6.919) ccw projected
  arc A622 (-14.1061, 13.7141) -> (-14.463, 13.8819) centre (-17.0087, 8.0015) ccw projected
  arc A623 (-13.8336, 13.5655) -> (-14.1061, 13.7141) centre (-16.4942, 9.0141) ccw projected
  arc A624 (-13.5655, 13.8336) -> (-13.8336, 13.5655) centre (0, 0) ccw projected
  arc A625 (-13.7141, 14.1061) -> (-13.5655, 13.8336) centre (-9.0141, 16.4942) ccw projected
  arc A626 (-13.8819, 14.463) -> (-13.7141, 14.1061) centre (-8.0015, 17.0087) ccw projected
  arc A627 (-14.0614, 14.9173) -> (-13.8819, 14.463) centre (-6.919, 17.4773) ccw projected
  arc A628 (-13.7681, 15.1885) -> (-14.0614, 14.9173) centre (0, 0) ccw projected
  arc A629 (-13.3293, 14.9739) -> (-13.7681, 15.1885) centre (-16.8806, 8.2689) ccw projected
  arc A630 (-12.9866, 14.7786) -> (-13.3293, 14.9739) centre (-16.3285, 9.3114) ccw projected
  arc A631 (-12.7266, 14.609) -> (-12.9866, 14.7786) centre (-15.7361, 10.2805) ccw projected
  arc A632 (-12.4383, 14.8553) -> (-12.7266, 14.609) centre (0, 0) ccw projected
  arc A633 (-12.5651, 15.1386) -> (-12.4383, 14.8553) centre (-7.6922, 17.1506) ccw projected
  arc A634 (-12.7043, 15.5076) -> (-12.5651, 15.1386) centre (-6.6424, 17.5841) ccw projected
  arc A635 (-12.8477, 15.9746) -> (-12.7043, 15.5076) centre (-5.5264, 17.9663) ccw projected
  arc A636 (-12.534, 16.2219) -> (-12.8477, 15.9746) centre (0, 0) ccw projected
  arc A637 (-12.1134, 15.9735) -> (-12.534, 16.2219) centre (-16.1798, 9.5679) ccw projected
  arc A638 (-11.7871, 15.752) -> (-12.1134, 15.9735) centre (-15.5476, 10.5638) ccw projected
  arc A639 (-11.5412, 15.5625) -> (-11.7871, 15.752) centre (-14.881, 11.4834) ccw projected
  arc A640 (-11.2344, 15.7854) -> (-11.5412, 15.5625) centre (0, 0) ccw projected
  arc A641 (-11.3386, 16.0778) -> (-11.2344, 15.7854) centre (-6.3229, 17.7012) ccw projected
  arc A642 (-11.4485, 16.4566) -> (-11.3386, 16.0778) centre (-5.2423, 18.051) ccw projected
  arc A643 (-11.5547, 16.9334) -> (-11.4485, 16.4566) centre (-4.0998, 18.3445) ccw projected
  arc A644 (-11.2226, 17.1553) -> (-11.5547, 16.9334) centre (0, 0) ccw projected
  arc A645 (-10.8227, 16.8747) -> (-11.2226, 17.1553) centre (-15.3792, 10.8078) ccw projected
  arc A646 (-10.5148, 16.6282) -> (-10.8227, 16.8747) centre (-14.6708, 11.7511) ccw projected
  arc A647 (-10.2846, 16.42) -> (-10.5148, 16.6282) centre (-13.9341, 12.6156) ccw projected
  arc A648 (-9.9612, 16.6182) -> (-10.2846, 16.42) centre (0, 0) ccw projected
  arc A649 (-10.0422, 16.9178) -> (-9.9612, 16.6182) centre (-4.9146, 18.1428) ccw projected
  arc A650 (-10.122, 17.3041) -> (-10.0422, 16.9178) centre (-3.8099, 18.4067) ccw projected
  arc A651 (-10.1905, 17.7877) -> (-10.122, 17.3041) centre (-2.6478, 18.6096) ccw projected
  arc A652 (-9.842, 17.9829) -> (-10.1905, 17.7877) centre (0, 0) ccw projected
  arc A653 (-9.4654, 17.6718) -> (-9.842, 17.9829) centre (-14.4838, 11.9812) ccw projected
  arc A654 (-9.1778, 17.4019) -> (-9.4654, 17.6718) centre (-13.7036, 12.8659) ccw projected
  arc A655 (-8.9646, 17.1763) -> (-9.1778, 17.4019) centre (-12.9014, 13.6699) ccw projected
  arc A656 (-8.6267, 17.3485) -> (-8.9646, 17.1763) centre (0, 0) ccw projected
  arc A657 (-8.6839, 17.6536) -> (-8.6267, 17.3485) centre (-3.476, 18.4724) ccw projected
  arc A658 (-8.7331, 18.0449) -> (-8.6839, 17.6536) centre (-2.3539, 18.6488) ccw projected
  arc A659 (-8.7635, 18.5324) -> (-8.7331, 18.0449) centre (-1.1796, 18.76) ccw projected
  arc A660 (-8.4007, 18.6997) -> (-8.7635, 18.5324) centre (0, 0) ccw projected
  arc A661 (-8.0497, 18.36) -> (-8.4007, 18.6997) centre (-13.4991, 13.0806) ccw projected
  arc A662 (-7.7842, 18.0684) -> (-8.0497, 18.36) centre (-12.6519, 13.9014) ccw projected
  arc A663 (-7.5893, 17.8267) -> (-7.7842, 18.0684) centre (-11.7891, 14.64) ccw projected
  arc A664 (-7.2389, 17.9719) -> (-7.5893, 17.8267) centre (0, 0) ccw projected
  arc A665 (-7.272, 18.2805) -> (-7.2389, 17.9719) centre (-2.0159, 18.6882) ccw projected
  arc A666 (-7.2904, 18.6745) -> (-7.272, 18.2805) centre (-0.8835, 18.776) ccw projected
  arc A667 (-7.2825, 19.1629) -> (-7.2904, 18.6745) centre (0.2959, 18.7947) ccw projected
  arc A668 (-6.9077, 19.3011) -> (-7.2825, 19.1629) centre (0, 0) ccw projected
  arc A669 (-6.5844, 18.9349) -> (-6.9077, 19.3011) centre (-12.4312, 14.0994) ccw projected
  arc A670 (-6.3425, 18.6234) -> (-6.5844, 18.9349) centre (-11.5222, 14.8512) ccw projected
  arc A671 (-6.1673, 18.3672) -> (-6.3425, 18.6234) centre (-10.6041, 15.5199) ccw projected
  arc A672 (-5.8066, 18.4844) -> (-6.1673, 18.3672) centre (0, 0) ccw projected
  arc A673 (-5.8154, 18.7947) -> (-5.8066, 18.4844) centre (-0.5434, 18.7888) ccw projected
  arc A674 (-5.8028, 19.1889) -> (-5.8154, 18.7947) centre (0.5924, 18.7875) ccw projected
  arc A675 (-5.7565, 19.6752) -> (-5.8028, 19.1889) centre (1.7696, 18.7136) ccw projected
  arc A676 (-5.372, 19.7836) -> (-5.7565, 19.6752) centre (0, 0) ccw projected
  arc A677 (-5.0785, 19.3932) -> (-5.372, 19.7836) centre (-11.2867, 15.0313) ccw projected
  arc A678 (-4.8618, 19.0636) -> (-5.0785, 19.3932) centre (-10.3215, 15.7095) ccw projected
  arc A679 (-4.7072, 18.7945) -> (-4.8618, 19.0636) centre (-9.3537, 16.304) ccw projected
  arc A680 (-4.3384, 18.883) -> (-4.7072, 18.7945) centre (0, 0) ccw projected
  arc A681 (-4.3228, 19.193) -> (-4.3384, 18.883) centre (0.9324, 18.7735) ccw projected
  arc A682 (-4.2793, 19.585) -> (-4.3228, 19.193) centre (2.0646, 18.6831) ccw projected
  arc A683 (-4.1951, 20.0662) -> (-4.2793, 19.585) centre (3.2324, 18.517) ccw projected
  arc A684 (-3.8033, 20.1441) -> (-4.1951, 20.0662) centre (0, 0) ccw projected
  arc A685 (-3.5413, 19.7318) -> (-3.8033, 20.1441) centre (-10.0726, 15.8705) ccw projected
  arc A686 (-3.3511, 19.3863) -> (-3.5413, 19.7318) centre (-9.0571, 16.4708) ccw projected
  arc A687 (-3.2181, 19.1059) -> (-3.3511, 19.3863) centre (-8.0457, 16.9876) ccw projected
  arc A688 (-2.8435, 19.1652) -> (-3.2181, 19.1059) centre (0, 0) ccw projected
  arc A689 (-2.8036, 19.473) -> (-2.8435, 19.1652) centre (2.4025, 18.6425) ccw projected
  arc A690 (-2.7295, 19.8604) -> (-2.8036, 19.473) centre (3.5241, 18.4635) ccw projected
  arc A691 (-2.6078, 20.3335) -> (-2.7295, 19.8604) centre (4.6753, 18.2064) ccw projected
  arc A692 (-2.2111, 20.3804) -> (-2.6078, 20.3335) centre (0, 0) ccw projected
  arc A693 (-1.9822, 19.9489) -> (-2.2111, 20.3804) centre (-8.7963, 16.6119) ccw projected
  arc A694 (-1.8197, 19.5895) -> (-1.9822, 19.9489) centre (-7.7369, 17.1307) ccw projected
  arc A695 (-1.7091, 19.2995) -> (-1.8197, 19.5895) centre (-6.6881, 17.5665) ccw projected
  arc A696 (-1.331, 19.3292) -> (-1.7091, 19.2995) centre (0, 0) ccw projected
  arc A697 (-1.2671, 19.633) -> (-1.331, 19.3292) centre (3.8577, 18.3965) ccw projected
  arc A698 (-1.1629, 20.0133) -> (-1.2671, 19.633) centre (4.9618, 18.1301) ccw projected
  arc A699 (-1.0044, 20.4754) -> (-1.1629, 20.0133) centre (6.0894, 17.7834) ccw projected
  arc A700 (-0.6052, 20.4911) -> (-1.0044, 20.4754) centre (0, 0) ccw projected
  arc A701 (-0.4109, 20.0429) -> (-0.6052, 20.4911) centre (-7.4658, 17.2508) ccw projected
  arc A702 (-0.2771, 19.6719) -> (-0.4109, 20.0429) centre (-6.369, 17.6849) ccw projected
  arc A703 (-0.1896, 19.3741) -> (-0.2771, 19.6719) centre (-5.2892, 18.0371) ccw projected
  arc A704 (0.1896, 19.3741) -> (-0.1896, 19.3741) centre (0, 0) ccw projected
  arc A705 (0.2771, 19.6719) -> (0.1896, 19.3741) centre (5.2892, 18.0371) ccw projected
  point P0 (-148.5, -105)
  point P1 (179.9715, 104.4715)
  point P2 (182.4715, 96.4715)
  point P3 (182.4715, 88.4715)
  point P4 (179.9715, 80.4715)
  point P5 (182.4715, 72.4715)
  point P6 (177.4715, 64.4715)
  point P7 (179.9715, 56.4715)
  point P8 (179.9715, 48.4715)
  point P9 (179.9715, 40.4715)
  point P10 (182.4715, 32.4715)
  point P11 (182.4715, 24.4715)
  point P12 (179.9715, 16.4715)
  point P13 (209.9715, 96.4715)
  point P14 (226.2215, 88.4715)
  point P15 (226.2215, 80.4715)
  point P16 (222.4715, 72.4715)
  point P17 (226.2215, 64.4715)
  point P18 (219.9715, 56.4715)
  point P19 (219.9715, 48.4715)
  point P20 (223.7215, 40.4715)
  point P21 (219.9715, 32.4715)
  point P22 (227.4715, 24.4715)
  point P23 (227.4715, 16.4715)
  point P24 (149.5, 125.9715)
  point P25 (149.5, 119.9715)
  point P26 (167.8125, 125.9715)
  point P27 (168.875, 119.9715)
  constraints: 128 point on circle, 64 centre point, 64 end point, 2 midpoint, 55 other
extrude "押し出し6" add sketch "スケッチ9" along normal blind 5 contours A1 A2 A63 A47 A46 A45 L15 A55 L7 A21 A22 A23 A62 A44 A43 A42 L14 A54 L16 L17 A48 L0 A0 | L17 L16 A50 L2 A6 A7 A8 A57 A29 A28 A27 L9 A49 L1 A3 A4 A5 A56 A26 A25 A24 L8 A48 | L17 A52 L4 A12 A13 A14 A59 A35 A34 A33 L11 A51 L3 A9 A10 A11 A58 A32 A31 A30 L10 A50 L16 | L16 A54 L6 A18 A19 A20 A61 A41 A40 A39 L13 A53 L5 A15 A16 A17 A60 A38 A37 A36 L12 A52 L17
sketch "スケッチ10" plane through (148.5, 105, 8) normal (0, 0, 1) x (1, 0, 0)
  arc A0 (0.8556, 4.3042) -> (0.5552, 3.8616) centre (2.0633, 3.1615) ccw projected
  arc A1 (2.0309, 5.0806) -> (0.8556, 4.3042) centre (3.1127, 2.1651) ccw projected
  arc A2 (2.1565, 5.0286) -> (2.0309, 5.0806) centre (0, 0) ccw projected
  arc A3 (2.4386, 3.6485) -> (2.1565, 5.0286) centre (-0.6701, 3.732) ccw projected
  arc A4 (2.338, 3.1232) -> (2.4386, 3.6485) centre (0.7765, 3.6944) ccw projected
  arc A5 (2.2731, 2.9935) -> (2.338, 3.1232) centre (1.787, 3.3179) ccw projected
  line L0 (2.2731, 2.9935) -> (1.9654, 2.5884) projected
  arc A6 (2.5884, 1.9654) -> (1.9654, 2.5884) centre (0, 0) ccw projected
  line L1 (2.5884, 1.9654) -> (2.9935, 2.2731) projected
  arc A7 (3.1232, 2.338) -> (2.9935, 2.2731) centre (3.3179, 1.787) ccw projected
  arc A8 (3.6485, 2.4386) -> (3.1232, 2.338) centre (3.6944, 0.7765) ccw projected
  arc A9 (5.0286, 2.1565) -> (3.6485, 2.4386) centre (3.732, -0.6701) ccw projected
  arc A10 (5.0806, 2.0309) -> (5.0286, 2.1565) centre (0, 0) ccw projected
  arc A11 (4.3042, 0.8556) -> (5.0806, 2.0309) centre (2.1651, 3.1127) ccw projected
  arc A12 (3.8616, 0.5552) -> (4.3042, 0.8556) centre (3.1615, 2.0633) ccw projected
  arc A13 (3.7241, 0.5094) -> (3.8616, 0.5552) centre (3.6097, 1.0825) ccw projected
  line L2 (3.7241, 0.5094) -> (3.22, 0.4405) projected
  arc A14 (3.22, -0.4405) -> (3.22, 0.4405) centre (0, 0) ccw projected
  line L3 (3.22, -0.4405) -> (3.7241, -0.5094) projected
  arc A15 (3.8616, -0.5552) -> (3.7241, -0.5094) centre (3.6097, -1.0825) ccw projected
  arc A16 (4.3042, -0.8556) -> (3.8616, -0.5552) centre (3.1615, -2.0633) ccw projected
  arc A17 (5.0806, -2.0309) -> (4.3042, -0.8556) centre (2.1651, -3.1127) ccw projected
  arc A18 (5.0286, -2.1565) -> (5.0806, -2.0309) centre (0, 0) ccw projected
  arc A19 (3.6485, -2.4386) -> (5.0286, -2.1565) centre (3.732, 0.6701) ccw projected
  arc A20 (3.1232, -2.338) -> (3.6485, -2.4386) centre (3.6944, -0.7765) ccw projected
  arc A21 (2.9935, -2.2731) -> (3.1232, -2.338) centre (3.3179, -1.787) ccw projected
  line L4 (2.9935, -2.2731) -> (2.5884, -1.9654) projected
  arc A22 (1.9654, -2.5884) -> (2.5884, -1.9654) centre (0, 0) ccw projected
  line L5 (1.9654, -2.5884) -> (2.2731, -2.9935) projected
  arc A23 (2.338, -3.1232) -> (2.2731, -2.9935) centre (1.787, -3.3179) ccw projected
  arc A24 (2.4386, -3.6485) -> (2.338, -3.1232) centre (0.7765, -3.6944) ccw projected
  arc A25 (2.1565, -5.0286) -> (2.4386, -3.6485) centre (-0.6701, -3.732) ccw projected
  arc A26 (2.0309, -5.0806) -> (2.1565, -5.0286) centre (0, 0) ccw projected
  arc A27 (0.8556, -4.3042) -> (2.0309, -5.0806) centre (3.1127, -2.1651) ccw projected
  arc A28 (0.5552, -3.8616) -> (0.8556, -4.3042) centre (2.0633, -3.1615) ccw projected
  arc A29 (0.5094, -3.7241) -> (0.5552, -3.8616) centre (1.0825, -3.6097) ccw projected
  line L6 (0.5094, -3.7241) -> (0.4405, -3.22) projected
  arc A30 (-0.4405, -3.22) -> (0.4405, -3.22) centre (0, 0) ccw projected
  line L7 (-0.4405, -3.22) -> (-0.5094, -3.7241) projected
  arc A31 (-0.5552, -3.8616) -> (-0.5094, -3.7241) centre (-1.0825, -3.6097) ccw projected
  arc A32 (-0.8556, -4.3042) -> (-0.5552, -3.8616) centre (-2.0633, -3.1615) ccw projected
  arc A33 (-2.0309, -5.0806) -> (-0.8556, -4.3042) centre (-3.1127, -2.1651) ccw projected
  arc A34 (-2.1565, -5.0286) -> (-2.0309, -5.0806) centre (0, 0) ccw projected
  arc A35 (-2.4387, -3.6513) -> (-2.1565, -5.0286) centre (0.6701, -3.732) ccw projected
  arc A36 (-2.338, -3.1232) -> (-2.4387, -3.6513) centre (-0.7765, -3.6944) ccw projected
  arc A37 (-2.2731, -2.9935) -> (-2.338, -3.1232) centre (-1.787, -3.3179) ccw projected
  line L8 (-2.2731, -2.9935) -> (-1.9654, -2.5884) projected
  arc A38 (-2.5884, -1.9654) -> (-1.9654, -2.5884) centre (0, 0) ccw projected
  line L9 (-2.5884, -1.9654) -> (-2.9935, -2.2731) projected
  arc A39 (-3.1232, -2.338) -> (-2.9935, -2.2731) centre (-3.3179, -1.787) ccw projected
  arc A40 (-3.6485, -2.4386) -> (-3.1232, -2.338) centre (-3.6944, -0.7765) ccw projected
  arc A41 (-5.0286, -2.1565) -> (-3.6485, -2.4386) centre (-3.732, 0.6701) ccw projected
  arc A42 (-5.0806, -2.0309) -> (-5.0286, -2.1565) centre (0, 0) ccw projected
  arc A43 (-4.3042, -0.8556) -> (-5.0806, -2.0309) centre (-2.1651, -3.1127) ccw projected
  arc A44 (-3.8616, -0.5552) -> (-4.3042, -0.8556) centre (-3.1615, -2.0633) ccw projected
  arc A45 (-3.7241, -0.5094) -> (-3.8616, -0.5552) centre (-3.6097, -1.0825) ccw projected
  line L10 (-3.7241, -0.5094) -> (-3.22, -0.4405) projected
  arc A46 (-3.22, 0.4405) -> (-3.22, -0.4405) centre (0, 0) ccw projected
  line L11 (-3.22, 0.4405) -> (-3.7241, 0.5094) projected
  arc A47 (-3.8616, 0.5552) -> (-3.7241, 0.5094) centre (-3.6097, 1.0825) ccw projected
  arc A48 (-4.3042, 0.8556) -> (-3.8616, 0.5552) centre (-3.1615, 2.0633) ccw projected
  arc A49 (-5.0806, 2.0309) -> (-4.3042, 0.8556) centre (-2.1651, 3.1127) ccw projected
  arc A50 (-5.0286, 2.1565) -> (-5.0806, 2.0309) centre (0, 0) ccw projected
  arc A51 (-3.6485, 2.4386) -> (-5.0286, 2.1565) centre (-3.732, -0.6701) ccw projected
  arc A52 (-3.1232, 2.338) -> (-3.6485, 2.4386) centre (-3.6944, 0.7765) ccw projected
  arc A53 (-2.9935, 2.2731) -> (-3.1232, 2.338) centre (-3.3179, 1.787) ccw projected
  line L12 (-2.9935, 2.2731) -> (-2.5884, 1.9654) projected
  arc A54 (-1.9654, 2.5884) -> (-2.5884, 1.9654) centre (0, 0) ccw projected
  line L13 (-1.9654, 2.5884) -> (-2.2731, 2.9935) projected
  arc A55 (-2.338, 3.1232) -> (-2.2731, 2.9935) centre (-1.787, 3.3179) ccw projected
  arc A56 (-2.4386, 3.6485) -> (-2.338, 3.1232) centre (-0.7765, 3.6944) ccw projected
  arc A57 (-2.1565, 5.0286) -> (-2.4386, 3.6485) centre (0.6701, 3.732) ccw projected
  arc A58 (-2.0309, 5.0806) -> (-2.1565, 5.0286) centre (0, 0) ccw projected
  arc A59 (-0.8556, 4.3042) -> (-2.0309, 5.0806) centre (-3.1127, 2.1651) ccw projected
  arc A60 (-0.5552, 3.8616) -> (-0.8556, 4.3042) centre (-2.0633, 3.1615) ccw projected
  arc A61 (-0.5094, 3.7241) -> (-0.5552, 3.8616) centre (-1.0825, 3.6097) ccw projected
  line L14 (-0.5094, 3.7241) -> (-0.4405, 3.22) projected
  arc A62 (0.4405, 3.22) -> (-0.4405, 3.22) centre (0, 0) ccw projected
  line L15 (0.4405, 3.22) -> (0.5094, 3.7241) projected
  arc A63 (0.5552, 3.8616) -> (0.5094, 3.7241) centre (1.0825, 3.6097) ccw projected
  point P0 (-148.5, -105)
hole "穴2" at (148.5, 105, 8) direction (0, 0, -1) diameter 4 end through all